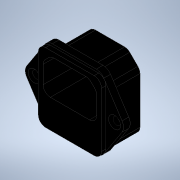
# Autodesk Inventor part: 719W-00 plug
Saved by Autodesk Inventor 2020 (Build 240168000, 168)
## iProperties
Created: 2020-04-10
Part Number: 719W-00 plug
Material: Generic
Document SubType Name: Modeling
Designer: angusaitken
Density: 1 g/cm^3
Appearance: Anodized - Black
Author: angusaitken
Autodesk Inventor part; units mm, degrees
ref_plane "YZ Plane" through (0, 0, 0) normal (1, 0, 0) x (0, 1, 0)
ref_plane "XZ Plane" through (0, 0, 0) normal (0, 1, 0) x (-1, 0, 0)
ref_plane "XY Plane" through (0, 0, 0) normal (0, 0, 1) x (1, 0, 0)
sketch "Sketch1" plane through (0, 0, 0) normal (0, 0, 1) x (1, 0, 0)
  line L0 (-22, -16.5) -> (22, -16.5)
  line L1 (22, -16.5) -> (22, 16.5)
  line L2 (22, 16.5) -> (-22, 16.5)
  line L3 (-22, 16.5) -> (-22, -16.5)
  line L4 (-22, -16.5) -> (22, 16.5) construction
  line L5 (22, -16.5) -> (-22, 16.5) construction
  line L6 (0, 0) -> (-18, 0)
  circle A0 centre (-18, 0) radius 4
  line L7 (0, 0) -> (-12, 0)
  line L8 (-12, 0) -> (-12, 16.5)
  line L9 (-12, 16.5) -> (-21.3489, 2.1875)
  line L10 (-21.3489, -2.1875) -> (-12, -16.5)
  line L11 (0, 16.5) -> (0, 9.3437)
  circle A1 centre (18, 0) radius 4
  line L12 (12, 16.5) -> (21.3489, 2.1875)
  line L13 (21.3489, -2.1875) -> (12, -16.5)
  dimension "d0" = 44
  dimension "d1" = 33
  dimension "d2" = 18
  dimension "d3" = 12
  constraints: 28 end point, 5 symmetric about line, 4 point on circle, 4 point on line, 3 midpoint, 2 centre point, 2 horizontal, 2 parallel, 2 perpendicular, 1 coincident, 1 tangent, 1 vertical, 1 other
  measures "d0" distance of L2.end L1.end
  measures "d1" distance of L1.end L0.end
  measures "d2" distance of L6.start L6.end
  measures "d3" distance of L6.start L7.end
extrude "Extrusion1" add sketch "Sketch1" along normal blind 3 contours L10 A0 L6 L8 L2 L12 A1 L13 L0 | A0 | L9 L8 L6 A0 | A1
fillet "Fillet1" radius 4 4 edges at (-12, 16.5, 1.5) (12, 16.5, 1.5) (12, -16.5, 1.5) (-12, -16.5, 1.5)
sketch "Sketch2" plane through (0, 0, 3) normal (0, 0, 1) x (1, 0, 0)
  line L0 (-10.9, -15.5) -> (10.9, -15.5)
  line L1 (14.15, -12.25) -> (14.15, 12.25)
  line L2 (10.9, 15.5) -> (-10.9, 15.5)
  line L3 (-14.15, 12.25) -> (-14.15, -12.25)
  line L4 (-14.15, -15.5) -> (14.15, 15.5) construction
  line L5 (14.15, -15.5) -> (-14.15, 15.5) construction
  arc A0 (-10.9, 15.5) -> (-14.15, 12.25) centre (-10.9, 12.25) ccw
  arc A1 (-14.15, -12.25) -> (-10.9, -15.5) centre (-10.9, -12.25) ccw
  arc A2 (10.9, -15.5) -> (14.15, -12.25) centre (10.9, -12.25) ccw
  arc A3 (14.15, 12.25) -> (10.9, 15.5) centre (10.9, 12.25) ccw
  point P0 (0, 0)
  dimension "d7" = 28.3
  dimension "d8" = 31
  dimension "d9" = 3.25
  dimension "d10" = 3.25
  constraints: 12 end point, 8 point on circle, 8 point on line, 8 tangent, 4 centre point, 2 equal radius, 2 midpoint, 2 parallel, 1 horizontal, 1 perpendicular
  measures "d7" distance of L5.end L4.end
  measures "d8" distance of L4.end L5.start
  measures "d9" radius of A0
  measures "d10" radius of A1
extrude "Extrusion2" add sketch "Sketch2" along normal blind 2
sketch "Sketch3" plane through (0, 0, 5) normal (0, 0, 1) x (1, 0, 0)
  line L0 (-12, -13.3) -> (12, -13.3)
  line L1 (12, -13.3) -> (12, 13.3)
  line L2 (12, 13.3) -> (-12, 13.3)
  line L3 (-12, 13.3) -> (-12, -13.3)
  line L4 (-12, -13.3) -> (12, 13.3) construction
  line L5 (12, -13.3) -> (-12, 13.3) construction
  line L6 (9.8351, 16.5) -> (-9.8351, 16.5) projected
  line L7 (-12, 13.3) -> (-12, -2.7)
  line L8 (-12, -2.7) -> (12, -2.7)
  line L9 (0, 13.3) -> (-8.5, 13.3)
  line L10 (-8.5, 13.3) -> (-12, 9.8)
  line L11 (0, 13.3) -> (0, 8.0839)
  line L12 (8.5, 13.3) -> (12, 9.8)
  point P0 (0, 0)
  dimension "d13" = 3.2
  dimension "d14" = 24
  dimension "d15" = 16
  dimension "d16" = 8.5
  dimension "d17" = 135
  constraints: 24 end point, 4 point on line, 3 midpoint, 2 parallel, 2 perpendicular, 2 symmetric about line, 1 horizontal, 1 vertical
  measures "d13" distance between parallel lines of L2 L6
  measures "d14" distance of L1.end L2.end
  measures "d15" distance of L2.end L7.end
  measures "d16" distance of L9.start L9.end
  measures "d17" angle of L10 L9
sketch "Sketch4" plane through (0, 0, 0) normal (0, 0, -1) x (-1, 0, 0)
  line L0 (-10.15, -15.5) -> (13.4, -15.5)
  line L1 (13.4, -15.5) -> (13.4, 15.5)
  line L2 (13.4, 15.5) -> (-13.4, 15.5)
  line L3 (-13.4, 15.5) -> (-13.4, -12.25)
  line L4 (-13.4, -15.5) -> (13.4, 15.5) construction
  line L5 (13.4, -15.5) -> (-13.4, 15.5) construction
  line L6 (-10.9, 15.5) -> (10.9, 15.5) projected
  line L7 (-7.8605, 15.5) -> (-13.4, 9.9605)
  line L8 (-7.8605, 15.5) -> (-0.0266, 15.5) construction
  arc A0 (-13.4, -12.25) -> (-10.15, -15.5) centre (-10.15, -12.25) ccw
  line L9 (-0.0266, 15.5) -> (-0.0266, 8.318)
  line L10 (7.8074, 15.5) -> (13.3469, 9.9605)
  arc A1 (10.0969, -15.5) -> (13.3469, -12.25) centre (10.0969, -12.25) ccw
  point P0 (0, 0)
  dimension "d18" = 26.8
  dimension "d19" = 31
  dimension "d20" = 135
  dimension "d21" = 3.25
  constraints: 20 end point, 5 symmetric about line, 4 point on circle, 4 point on line, 2 centre point, 2 horizontal, 2 midpoint, 2 parallel, 2 tangent, 1 equal length, 1 perpendicular, 1 vertical, 1 other
  measures "d18" distance of L2.end L1.end
  measures "d19" distance of L1.end L0.end
  measures "d20" angle of L7 L8
  measures "d21" radius of A0
extrude "Extrusion3" add sketch "Sketch4" along normal blind 13 contours A0 L3 L7 L2 L1 L0
fillet "Fillet2" radius 3.25 1 edges at (-13.4, -15.5, -6.5)
sketch "Sketch5" plane through (0, 0, -13) normal (0, 0, -1) x (-1, 0, 0)
  line L0 (-13.4, -12.25) -> (-13.4, 9.9605) projected
  line L1 (-13.4, 9.9605) -> (13.4, 9.9605)
  line L2 (13.4, 14.3567) -> (13.4, -12.25) projected
  line L3 (13.4, 9.9605) -> (7.8605, 15.5)
  line L4 (-7.8605, 15.5) -> (12.4808, 15.5) projected
  line L5 (13.4, 9.9605) -> (21.234, 9.9605) construction
  line L6 (10.8633, 12.4973) -> (4.8774, 18.4831)
  line L7 (4.8774, 18.4831) -> (17.0943, 6.2662)
  point P0 (0, 0)
  dimension "d25" = 135
  constraints: 10 end point, 4 point on line, 2 horizontal, 1 equal length
  measures "d25" angle of L5 L3
chamfer "Chamfer1" distance 5.5 angle 45 1 edges at (-13.4, 15.5, -6.5)
extrude "Extrusion4" cut sketch "Sketch3" against normal blind 16.175 contours L3 L10 L2 L12 L1 L8
fillet "Fillet3" radius 3.25 6 edges at (12, -2.7, -3.0875) (12, 9.8, -3.0875) (8.5, 13.3, -3.0875) (-8.5, 13.3, -3.0875) (-12, 9.8, -3.0875) (-12, -2.7, -3.0875)
sketch "Sketch6" plane through (0, 0, 3) normal (0, 0, 1) x (1, 0, 0)
  arc A0 (-21.3489, 2.1875) -> (-21.3489, -2.1875) centre (-18, 0) ccw projected
  arc A1 (21.3489, -2.1875) -> (21.3489, 2.1875) centre (18, 0) ccw projected
  circle A2 centre (-18, 0) radius 1.7
  circle A3 centre (18, 0) radius 1.7
  point P0 (0, 0)
  dimension "d32" = 3.4
  dimension "d33" = 3.4
  constraints: 2 centre point, 2 coincident
  measures "d32" diameter of A2
  measures "d33" diameter of A3
hole "Hole1" at (-18, 0, 3) at (18, 0, 3) direction (0, 0, -1) diameter 3.4 end through all
chamfer "Chamfer2" distance 1 angle 45 2 edges at (-18, 1.7, 3) (18, 1.7, 3)
fillet "Fillet4" radius 3.25 4 edges at (13.4, 9.9605, -6.5) (7.8605, 15.5, -6.5) (-7.9, 15.5, -6.5) (-13.4, 10, -6.5)
body "Solid1"
